Autodesk Fusion 360 part; units mm, degrees
(part 2 of 2)
  spline S127 degree 3 poles (-34.1268, -62.7988) (-34.0437, -63.0573) (-33.9603, -63.3031) (-33.9415, -63.3451) knots 0 0 0 0 1 1 1 1
  spline S128 degree 3 poles (-33.9415, -63.3451) (-33.803, -63.6544) (-32.8286, -66.7708) (-32.7158, -67.2652) knots 0 0 0 0 1 1 1 1
  spline S129 degree 3 poles (-32.7158, -67.2652) (-32.6807, -67.4192) (-32.621, -67.6435) (-32.5832, -67.7637) knots 0 0 0 0 1 1 1 1
  spline S130 degree 3 poles (-32.5832, -67.7637) (-32.3971, -68.3547) (-32.3528, -68.8591) (-32.3336, -70.5999) knots 0 0 0 0 1 1 1 1
  spline S131 degree 3 poles (-32.3336, -70.5999) (-32.3231, -71.5519) (-32.2931, -72.4912) (-32.2668, -72.6872) knots 0 0 0 0 1 1 1 1
  spline S132 degree 3 poles (-32.2668, -72.6872) (-32.1806, -73.3314) (-32.117, -73.9983) (-32.0606, -74.8509) knots 0 0 0 0 1 1 1 1
  spline S133 degree 3 poles (-32.0606, -74.8509) (-31.9829, -76.0238) (-31.7879, -77.4944) (-31.6454, -77.9819) knots 0 0 0 0 1 1 1 1
  spline S134 degree 3 poles (-31.6454, -77.9819) (-31.436, -78.6986) (-31.2739, -79.0012) (-30.6096, -79.9165) knots 0 0 0 0 1 1 1 1
  spline S135 degree 3 poles (-30.6096, -79.9165) (-29.5815, -81.3329) (-29.377, -81.6216) (-29.1145, -82.0279) knots 0 0 0 0 1 1 1 1
  spline S136 degree 3 poles (-29.1145, -82.0279) (-28.6226, -82.789) (-28.5899, -82.8625) (-28.7211, -82.9129) knots 0 0 0 0 1 1 1 1
  spline S137 degree 3 poles (-28.7211, -82.9129) (-28.7913, -82.9398) (-29.1714, -82.6451) (-29.74, -82.1228) knots 0 0 0 0 1 1 1 1
  spline S138 degree 3 poles (-29.74, -82.1228) (-29.852, -82.0199) (-30.0041, -81.8884) (-30.078, -81.8305) knots 0 0 0 0 1 1 1 1
  spline S139 degree 3 poles (-30.078, -81.8305) (-30.1519, -81.7727) (-30.3346, -81.5745) (-30.4842, -81.3903) knots 0 0 0 0 1 1 1 1
  spline S140 degree 3 poles (-30.4842, -81.3903) (-30.6337, -81.206) (-30.7642, -81.0798) (-30.7742, -81.1099) knots 0 0 0 0 1 1 1 1
  spline S141 degree 3 poles (-30.7742, -81.1099) (-30.822, -81.2532) (-29.9655, -82.5432) (-29.6399, -82.8184) knots 0 0 0 0 1 1 1 1
  spline S142 degree 3 poles (-29.6399, -82.8184) (-29.6067, -82.8464) (-29.5386, -82.9323) (-29.4885, -83.0093) knots 0 0 0 0 1 1 1 1
  spline S143 degree 3 poles (-29.4885, -83.0093) (-29.399, -83.1467) (-29.3993, -83.1493) (-29.5062, -83.1493) knots 0 0 0 0 1 1 1 1
  spline S144 degree 3 poles (-29.5062, -83.1493) (-29.5986, -83.1493) (-29.828, -82.973) (-30.1699, -82.6392) knots 0 0 0 0 1 1 1 1
  spline S145 degree 3 poles (-30.1699, -82.6392) (-30.6146, -82.205) (-31.1212, -81.4552) (-31.4236, -80.7839) knots 0 0 0 0 1 1 1 1
  spline S146 degree 3 poles (-31.4236, -80.7839) (-31.6038, -80.3839) (-31.7009, -80.2532) (-31.6995, -80.4128) knots 0 0 0 0 1 1 1 1
  spline S147 degree 3 poles (-31.6995, -80.4128) (-31.6985, -80.5293) (-31.3408, -81.49) (-31.214, -81.7168) knots 0 0 0 0 1 1 1 1
  spline S148 degree 3 poles (-31.214, -81.7168) (-31.0652, -81.983) (-31.0566, -82.0802) (-31.1817, -82.0802) knots 0 0 0 0 1 1 1 1
  spline S149 degree 3 poles (-31.1817, -82.0802) (-31.3966, -82.0802) (-32.2108, -80.6413) (-32.4925, -79.7637) knots 0 0 0 0 1 1 1 1
  spline S150 degree 3 poles (-32.4925, -79.7637) (-32.6107, -79.3954) (-32.6798, -79.3466) (-32.7086, -79.611) knots 0 0 0 0 1 1 1 1
  spline S151 degree 3 poles (-32.7086, -79.611) (-32.7312, -79.819) (-32.8325, -79.9223) (-32.9157, -79.8222) knots 0 0 0 0 1 1 1 1
  spline S152 degree 3 poles (-32.9157, -79.8222) (-32.97, -79.7566) (-33.3975, -78.6018) (-33.465, -78.3382) knots 0 0 0 0 1 1 1 1
  spline S153 degree 3 poles (-33.465, -78.3382) (-33.5156, -78.1402) (-33.6593, -77.9046) (-33.7461, -77.877) knots 0 0 0 0 1 1 1 1
  spline S154 degree 3 poles (-33.7461, -77.877) (-33.8361, -77.8484) (-34.2273, -77.2842) (-34.3392, -77.0216) knots 0 0 0 0 1 1 1 1
  spline S155 degree 3 poles (-34.3392, -77.0216) (-34.3734, -76.9414) (-34.4157, -76.6207) (-34.4332, -76.3088) knots 0 0 0 0 1 1 1 1
  spline S156 degree 3 poles (-34.4332, -76.3088) (-34.465, -75.7428) (-34.4654, -75.7414) (-34.6584, -75.521) knots 0 0 0 0 1 1 1 1
  spline S157 degree 3 poles (-34.6584, -75.521) (-34.9653, -75.1705) (-35.0614, -74.9202) (-35.1055, -74.3574) knots 0 0 0 0 1 1 1 1
  spline S158 degree 3 poles (-35.1055, -74.3574) (-35.1424, -73.887) (-35.1584, -73.8345) (-35.3825, -73.4497) knots 0 0 0 0 1 1 1 1
  spline S159 degree 3 poles (-35.3825, -73.4497) (-35.5422, -73.1755) (-35.6595, -72.8866) (-35.7394, -72.5708) knots 0 0 0 0 1 1 1 1
  spline S160 degree 3 poles (-35.7394, -72.5708) (-35.8064, -72.3056) (-35.9039, -72.0506) (-35.9628, -71.9865) knots 0 0 0 0 1 1 1 1
  spline S161 degree 3 poles (-35.9628, -71.9865) (-36.1469, -71.7858) (-36.3726, -71.3718) (-36.4564, -71.081) knots 0 0 0 0 1 1 1 1
  spline S162 degree 3 poles (-36.4564, -71.081) (-36.5198, -70.8611) (-36.5861, -70.7582) (-36.7558, -70.6163) knots 0 0 0 0 1 1 1 1
  spline S163 degree 3 poles (-36.7558, -70.6163) (-37.0892, -70.3376) (-37.2544, -69.9769) (-37.2879, -69.4544) knots 0 0 0 0 1 1 1 1
  spline S164 degree 3 poles (-37.2879, -69.4544) (-37.3097, -69.1147) (-37.3425, -68.979) (-37.4404, -68.8234) knots 0 0 0 0 1 1 1 1
  spline S165 degree 3 poles (-37.4404, -68.8234) (-37.6835, -68.4373) (-38.0129, -67.7032) (-38.0129, -67.5475) knots 0 0 0 0 1 1 1 1
  spline S166 degree 3 poles (-38.0129, -67.5475) (-38.0129, -67.4382) (-38.0926, -67.2806) (-38.272, -67.0347) knots 0 0 0 0 1 1 1 1
  spline S167 degree 3 poles (-38.272, -67.0347) (-38.6192, -66.559) (-38.7257, -66.3033) (-38.7257, -65.9452) knots 0 0 0 0 1 1 1 1
  spline S168 degree 3 poles (-38.7257, -65.9452) (-38.7257, -65.7111) (-38.7474, -65.6323) (-38.8333, -65.5549) knots 0 0 0 0 1 1 1 1
  spline S169 degree 3 poles (-38.8333, -65.5549) (-39.0112, -65.3946) (-39.2508, -64.8306) (-39.2564, -64.5588) knots 0 0 0 0 1 1 1 1
  spline S170 degree 3 poles (-39.2564, -64.5588) (-39.2608, -64.3462) (-39.2879, -64.2881) (-39.4714, -64.0976) knots 0 0 0 0 1 1 1 1
  spline S171 degree 3 poles (-39.4714, -64.0976) (-39.9128, -63.6393) (-40.1267, -63.115) (-40.0352, -62.7154) knots 0 0 0 0 1 1 1 1
  spline S172 degree 3 poles (-40.0352, -62.7154) (-39.9868, -62.5036) (-39.9929, -62.4754) (-40.1208, -62.3234) knots 0 0 0 0 1 1 1 1
  spline S173 degree 3 poles (-40.1208, -62.3234) (-40.4603, -61.9201) (-40.6072, -61.4176) (-40.5108, -60.9904) knots 0 0 0 0 1 1 1 1
  spline S174 degree 3 poles (-40.5108, -60.9904) (-40.4596, -60.7636) (-40.4651, -60.7362) (-40.5978, -60.553) knots 0 0 0 0 1 1 1 1
  spline S175 degree 3 poles (-40.5978, -60.553) (-40.6757, -60.4455) (-40.78, -60.268) (-40.8296, -60.1585) knots 0 0 0 0 1 1 1 1
  spline S176 degree 3 poles (-40.8296, -60.1585) (-40.8919, -60.0213) (-41.0256, -59.8845) (-41.261, -59.7174) knots 0 0 0 0 1 1 1 1
  spline S177 degree 3 poles (-41.261, -59.7174) (-42.0881, -59.1303) (-44.2964, -57.5064) (-44.5077, -57.3299) knots 0 0 0 0 1 1 1 1
  spline S178 degree 3 poles (-44.5077, -57.3299) (-44.5863, -57.2642) (-44.7437, -57.1277) (-44.8574, -57.0266) knots 0 0 0 0 1 1 1 1
  spline S179 degree 3 poles (-44.8574, -57.0266) (-44.971, -56.9255) (-45.2898, -56.667) (-45.5657, -56.4522) knots 0 0 0 0 1 1 1 1
  line L14 (-45.5657, -56.4522) -> (-46.0675, -56.0617)
  line L15 (-46.0675, -56.0617) -> (-46.4312, -56.0891)
  spline S180 degree 3 poles (-46.4312, -56.0891) (-46.9252, -56.1264) (-50.0446, -56.2089) (-52.3442, -56.2455) knots 0 0 0 0 1 1 1 1
  spline S181 degree 3 poles (-52.3442, -56.2455) (-53.3803, -56.262) (-54.7777, -56.3092) (-55.4498, -56.3505) knots 0 0 0 0 1 1 1 1
  spline S182 degree 3 poles (-55.4498, -56.3505) (-56.3967, -56.4086) (-57.6164, -56.4222) (-60.8717, -56.4107) knots 0 0 0 0 1 1 1 1
  spline S183 degree 3 poles (-60.8717, -56.4107) (-66.3285, -56.3914) (-67.7406, -56.4019) (-68.4792, -56.4669) knots 0 0 0 0 1 1 1 1
  spline S184 degree 3 poles (-68.4792, -56.4669) (-68.971, -56.5102) (-69.1791, -56.5059) (-69.5737, -56.444) knots 0 0 0 0 1 1 1 1
  spline S185 degree 3 poles (-69.5737, -56.444) (-70.179, -56.3491) (-70.3024, -56.3006) (-70.494, -56.0823) knots 0 0 0 0 1 1 1 1
  spline S186 degree 3 poles (-70.494, -56.0823) (-70.6855, -55.8643) (-70.6913, -55.6678) (-70.5128, -55.4557) knots 0 0 0 0 1 1 1 1
  spline S187 degree 3 poles (-24.1416, -39.57) (-24.1286, -39.57) (-24.0905, -39.5184) (-24.0569, -39.4554) knots 0 0 0 0 1 1 1 1
  spline S188 degree 3 poles (-24.0569, -39.4554) (-24.0016, -39.3516) (-24.0038, -39.3474) (-24.0806, -39.4107) knots 0 0 0 0 1 1 1 1
  spline S189 degree 3 poles (-24.0806, -39.4107) (-24.1595, -39.4758) (-24.1956, -39.57) (-24.1416, -39.57) knots 0 0 0 0 1 1 1 1
extrude "Extrusion6" [suppressed]
extrude "Extrusion1" [suppressed]
extrude "Extrusion2" [suppressed]
sketch "Skizze2" plane through (0, 0, 2) normal (0, 0, 1) x (-1, 0, 0)
  line L0 (0, -109) -> (0, 0)
  line L1 (0, 0) -> (-85, 0)
  line L2 (-85, 0) -> (-85, -109)
  line L3 (-85, -109) -> (0, -109)
  circle A0 centre (-42.5, -54.5) radius 35
  circle A1 centre (-42.5, -89.5) radius 15
  circle A2 centre (-42.5, -19.5) radius 15
  dimension "d27" = 70
  dimension "d28" = 54.5
  dimension "d29" = 42.5
  dimension "d30" = 30
  dimension "d31" = 30
  dimension "d32" = 42.5
  dimension "d33" = 19.5
  dimension "d34" = 19.5
  constraint coincident A0 A1.centre
  constraint coincident A0 A2.centre
  measures "d27" diameter of A0
  measures "d28" distance of L1 A0.centre
  measures "d29" distance of L0 A0.centre
  measures "d30" diameter of A1
  measures "d31" diameter of A2
  measures "d32" distance of L2 A0.centre
  measures "d33" distance of L3 A1.centre
  measures "d34" distance of L1 A2.centre
equation "d28 = ( 109 / 2 ) * 1 mm"
equation "d29 = ( 85 / 2 ) * 1 mm"
equation "d40 = ( 85 / 2 ) * 1 mm"
